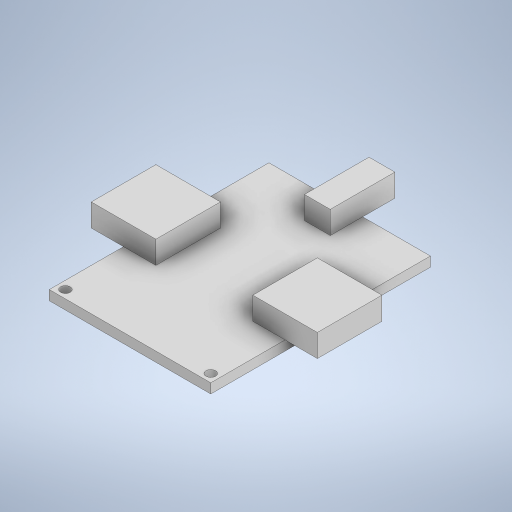
# Autodesk Inventor part: Holybro PM07 PowerDistributionBoard
Saved by Autodesk Inventor 2023 (Build 270158000, 158)
## iProperties
Created: 2022-12-11
Part Number: Holybro PM07 PowerDistributionBoard
Material: Generic
Document SubType Name: Modeling
Designer: Administrator
Density: 1 g/cm^3
Appearance: Default
Author: Administrator
Autodesk Inventor part; units mm, degrees
ref_plane "YZ Plane" through (0, 0, 0) normal (1, 0, 0) x (0, 1, 0)
ref_plane "XZ Plane" through (0, 0, 0) normal (0, 1, 0) x (-1, 0, 0)
ref_plane "XY Plane" through (0, 0, 0) normal (0, 0, 1) x (1, 0, 0)
sketch "Sketch1" plane through (0, 0, 0) normal (0, 1, 0) x (-1, 0, 0)
  line L0 (0, 0) -> (45, 0) construction
  line L1 (45, 0) -> (45, -45) construction
  line L2 (45, -45) -> (0, -45) construction
  line L3 (0, -45) -> (0, 0) construction
  circle A0 centre (45, 0) radius 1.5
  circle A1 centre (45, -45) radius 1.5
  circle A2 centre (0, -45) radius 1.5
  circle A3 centre (0, 0) radius 1.5
  line L4 (-2.5, 2.5) -> (47.5, 2.5)
  line L5 (47.5, 2.5) -> (47.5, -65.5)
  line L6 (47.5, -65.5) -> (-2.5, -65.5)
  line L7 (-2.5, -65.5) -> (-2.5, 2.5)
  dimension "d0" = 45
  dimension "d1" = 45
  dimension "d2" = 3
  dimension "d3" = 3
  dimension "d4" = 3
  dimension "d5" = 3
  dimension "d6" = 50
  dimension "d7" = 68
  dimension "d8" = 2.5
  dimension "d9" = 2.5
  constraints: 16 end point, 4 centre point, 4 coincident, 4 parallel, 2 horizontal, 2 perpendicular
  measures "d0" distance of L1.end L2.end
  measures "d1" distance of L0.end L1.end
  measures "d2" diameter of A0
  measures "d3" diameter of A1
  measures "d4" diameter of A2
  measures "d5" diameter of A3
  measures "d6" distance of L5.end L6.end
  measures "d7" distance of L4.end L5.end
  measures "d8" distance from line of L2.end L7
  measures "d9" distance from line of L0.start L4
extrude "Extrusion1" add sketch "Sketch1" along normal blind 3
sketch "Sketch2" plane through (0, 3, 0) normal (0, 1, 0) x (1, 0, 0)
  line L0 (2.5, -2.5) -> (2.5, 65.5) projected
  line L1 (2.5, 40.5) -> (-7.5, 40.5)
  line L2 (-7.5, 40.5) -> (-7.5, 20.5)
  line L3 (-7.5, 20.5) -> (2.5, 20.5)
  line L4 (2.5, 20.5) -> (2.5, 40.5)
  line L5 (2.5, 65.5) -> (-47.5, 65.5) projected
  line L6 (-47.5, 65.5) -> (-47.5, -2.5) projected
  line L7 (-47.5, 40.5) -> (-37.5, 40.5)
  line L8 (-37.5, 40.5) -> (-37.5, 20.5)
  line L9 (-37.5, 20.5) -> (-47.5, 20.5)
  line L10 (-47.5, 20.5) -> (-47.5, 40.5)
  line L11 (-26.5, 65.5) -> (-18.5, 65.5)
  line L12 (-18.5, 65.5) -> (-18.5, 55.5)
  line L13 (-18.5, 55.5) -> (-26.5, 55.5)
  line L14 (-26.5, 55.5) -> (-26.5, 65.5)
  point P0 (0, 0)
  point P1 (2.5, 20.5)
  dimension "d12" = 10
  dimension "d13" = 20
  dimension "d14" = 25
  dimension "d15" = 10
  dimension "d16" = 20
  dimension "d19" = 8
  dimension "d20" = 10
  dimension "d21" = 50
  dimension "d22" = 68
  dimension "d23" = 21
  constraints: 24 end point, 6 parallel, 3 horizontal, 3 perpendicular, 3 point on line
  measures "d12" distance of L3.end L2.end
  measures "d13" distance of L2.end L1.end
  measures "d14" distance between parallel lines of L5 L1
  measures "d15" distance of L8.end L9.end
  measures "d16" distance of L7.end L8.end
  measures "d19" distance of L12.end L13.end
  measures "d20" distance of L11.end L12.end
  measures "d21" distance between parallel lines of L0 L6
  measures "d22" distance of L5.end L6.end
  measures "d23" distance between parallel lines of L6 L14
extrude "Extrusion2" add sketch "Sketch2" along normal blind 7
sketch "Sketch3" plane through (2.5, 0, 2.5) normal (1, 0, 0) x (0, 0, -1)
  line L0 (43, 10) -> (23, 10) projected
  line L1 (43, 3) -> (23, 3) projected
  line L2 (23, 10) -> (43, 10)
  line L3 (43, 10) -> (43, 3)
  line L4 (43, 3) -> (23, 3)
  line L5 (23, 3) -> (23, 10)
  point P0 (2.5, 0)
  constraints: 8 end point, 2 parallel, 1 horizontal, 1 perpendicular
extrude "Extrusion3" add sketch "Sketch3" along normal blind 10
sketch "Sketch4" plane through (-47.5, 0, -65.5) normal (-1, 0, 0) x (0, 0, 1)
  line L0 (25, 3) -> (25, 10) projected
  line L1 (45, 3) -> (45, 10) projected
  line L2 (25, 10) -> (45, 10)
  line L3 (45, 10) -> (45, 3)
  line L4 (45, 3) -> (25, 3)
  line L5 (25, 3) -> (25, 10)
  point P0 (65.5, 0)
  constraints: 8 end point, 2 parallel, 1 horizontal, 1 perpendicular
extrude "Extrusion4" add sketch "Sketch4" along normal blind 10
sketch "Sketch5" plane through (2.5, 0, -65.5) normal (0, 0, -1) x (-1, 0, 0)
  line L0 (21, 10) -> (29, 10) projected
  line L1 (29, 3) -> (50, 3) projected
  line L2 (21, 10) -> (29, 10)
  line L3 (29, 10) -> (29, 3)
  line L4 (29, 3) -> (21, 3)
  line L5 (21, 3) -> (21, 10)
  point P0 (2.5, 0)
  constraints: 8 end point, 2 parallel, 1 horizontal, 1 perpendicular
extrude "Extrusion5" add sketch "Sketch5" along normal blind 10
equation "\"d8\" = -0.5 * d0 + 0.5 * d6"
equation "\"d9\" = d8"
equation "\"d23\" = -0.5 * d19 + 0.5 * d21"
body "Solid1"
